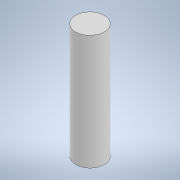
# Autodesk Inventor part: Peg
Saved by Autodesk Inventor 2020.2 (Build 242310000, 310)
## iProperties
Created: 2020-04-17
Part Number: Peg
Material: Generic
Document SubType Name: Modeling
Designer: Tanana
Density: 1 g/cm^3
Appearance: Default
Author: Tanana
Autodesk Inventor part; units mm, degrees
ref_plane "YZ Plane" through (0, 0, 0) normal (1, 0, 0) x (0, 1, 0)
ref_plane "XZ Plane" through (0, 0, 0) normal (0, 1, 0) x (-1, 0, 0)
ref_plane "XY Plane" through (0, 0, 0) normal (0, 0, 1) x (1, 0, 0)
sketch "Sketch1" plane through (0, 0, 0) normal (0, 1, 0) x (-1, 0, 0)
  circle A0 centre (14.5143, 15.8504) radius 12.7
  circle A1 centre (14.5143, 15.8504) radius 12.7
  point P0 (0, 0)
  dimension "d0" = 25.4
  constraints: 2 centre point, 1 coincident, 1 concentric
  measures "d0" diameter of A0
extrude "Extrusion1" add sketch "Sketch1" along normal blind 101.6
body "Solid1"
